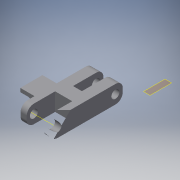
# Autodesk Inventor part: lever2
Saved by Autodesk Inventor 2016 (Build 200138000, 138)
## iProperties
Created: 2015-09-30
Part Number: lever2
Material: Generic
Document SubType Name: Modeling
Designer: Jesse Stevenson
Density: 1 g/cm^3
Appearance: Default
Author: Jesse Stevenson
Autodesk Inventor part; units mm, degrees
ref_plane "YZ Plane" through (0, 0, 0) normal (1, 0, 0) x (0, 1, 0)
ref_plane "XZ Plane" through (0, 0, 0) normal (0, 1, 0) x (-1, 0, 0)
ref_plane "XY Plane" through (0, 0, 0) normal (0, 0, 1) x (1, 0, 0)
ref_plane "Work Plane1" through (8.001, 26.0985, -18.0717) normal (0, 1, 0) x (0, 0, -1)
sketch "Sketch1" plane through (8.001, 26.0985, -18.0717) normal (0, 1, 0) x (0, 0, -1)
  line L0 (-43.7282, -1.4601) -> (-43.7282, -1.8842)
  line L1 (-43.7282, -1.8842) -> (-9.3098, -1.8842)
  line L2 (-9.3098, -1.8842) -> (-9.3098, 2.815)
  line L3 (-43.7282, 11.0271) -> (-43.7282, 11.4512)
  line L4 (-43.7282, 11.4512) -> (-9.3098, 11.4512)
  line L5 (-9.3098, 11.4512) -> (-9.3098, 6.752)
  line L6 (-43.7282, -1.4601) -> (-43.7282, 11.0271)
  line L7 (-9.3098, 2.815) -> (-25.0363, 2.815)
  line L8 (-25.0363, 2.815) -> (-25.0363, 6.752)
  line L9 (-25.0363, 6.752) -> (-9.3098, 6.752)
  line L10 (-18.0537, 2.815) -> (-18.0537, -1.8842) construction
  line L11 (-18.0537, 6.752) -> (-18.0537, 11.4512) construction
  line L12 (-16.6851, 3.45) -> (-16.6851, 6.117) construction
  line L13 (-16.6851, 3.45) -> (-12.9069, 3.45) construction
  line L14 (-12.9069, 3.45) -> (-12.9069, 6.117) construction
  line L15 (-12.9069, 6.117) -> (-16.6851, 6.117) construction
  point P0 (-18.0717, 8.001)
  dimension "d19" = 0.635
  dimension "d20" = 0.635
  constraints: 24 end point, 6 point on line, 4 collinear, 3 parallel, 3 perpendicular, 2 horizontal
  measures "d19" distance between parallel lines of L7 L13
  measures "d20" distance between parallel lines of L9 L15
extrude "Extrusion1" add sketch "Sketch1" along normal blind 7.9375
sketch "Sketch2" plane through (9.8852, 26.0985, 25.6565) normal (1, 0, 0) x (0, 0, -1)
  line L0 (34.4184, 0) -> (0, 0) construction
  line L1 (34.4184, 0) -> (34.4184, 7.9375) construction
  line L2 (0, 7.9375) -> (34.4184, 7.9375) construction
  line L3 (0, 0) -> (0, 7.9375) construction
  line L4 (34.4184, 0) -> (34.4184, 7.9375) construction
  line L5 (34.4184, 3.9687) -> (0, 3.9687) construction
  line L6 (34.4184, 0) -> (0, 0) construction
  line L7 (28.9311, 0) -> (28.9311, 7.9375) construction
  line L8 (34.4184, 7.9375) -> (14.8298, 7.9375) construction
  circle A0 centre (28.9311, 3.9687) radius 1.7859
  point P0 (25.6565, -26.0985)
  dimension "d8" = 3.5719
  constraints: 4 end point, 3 midpoint, 3 point on line, 1 centre point, 1 perpendicular
  measures "d8" diameter of A0
extrude "Extrusion2" cut sketch "Sketch2" against normal through all
fillet "Fillet1" radius 3.175 2 edges at (3.2175, 34.036, 25.6565) (3.2175, 26.0985, 25.6565)
sketch "Sketch3" plane through (9.8852, 26.0985, -8.7619) normal (1, 0, 0) x (0, 0, -1)
  circle A0 centre (-5.4873, 3.9688) radius 1.7859 projected
  line L0 (0, 0) -> (-31.2434, 0) projected
  line L1 (0, 0) -> (0, 7.9375) projected
  line L2 (-31.2434, 7.9375) -> (0, 7.9375) projected
  line L3 (-34.4184, 3.175) -> (-34.4184, 4.7625) projected
  line L4 (-31.2434, 3.175) -> (-31.2434, 4.7625) construction
  circle A1 centre (-31.2434, 3.9687) radius 1.7859
  arc A2 (-34.4184, 3.175) -> (-31.2434, 0) centre (-31.2434, 3.175) ccw projected
  arc A3 (-31.2434, 7.9375) -> (-34.4184, 4.7625) centre (-31.2434, 4.7625) ccw projected
  point P0 (-8.7619, -26.0985)
  dimension "d7" = 3.5719
  constraints: 2 end point, 1 centre point, 1 midpoint, 1 vertical
  measures "d7" diameter of A1
extrude "Extrusion3" cut sketch "Sketch3" against normal through all contours A1
sketch "Sketch5" plane through (9.8852, 26.0985, -8.7619) normal (1, 0, 0) x (0, 0, -1)
  circle A0 centre (-31.2434, 3.9688) radius 1.7859 construction
  circle A1 centre (-5.4873, 3.9688) radius 1.7859 construction
  line L0 (0, 0) -> (-31.2434, 0) construction
  line L1 (0, 0) -> (0, 7.9375) construction
  line L2 (-31.2434, 7.9375) -> (0, 7.9375) construction
  line L3 (-34.4184, 3.175) -> (-34.4184, 4.7625) construction
  line L4 (-15.9544, 0) -> (0, 0) projected
  line L5 (-2.2351, 0) -> (-2.2351, 7.9375)
  line L6 (-15.9544, 7.9375) -> (0, 7.9375) projected
  line L7 (-2.2351, 0) -> (-8.7527, 0)
  line L8 (-34.4184, 7.9375) -> (0, 7.9375) projected
  line L9 (-2.2351, 0) -> (0, 0)
  line L10 (0, 0) -> (0, 7.9375)
  line L11 (0, 7.9375) -> (-2.2351, 7.9375)
  line L12 (-2.2351, 7.9375) -> (-2.2351, 0)
  arc A2 (-34.4184, 3.175) -> (-31.2434, 0) centre (-31.2434, 3.175) ccw projected
  arc A3 (-31.2434, 7.9375) -> (-34.4184, 4.7625) centre (-31.2434, 4.7625) ccw projected
  point P0 (-8.7619, -26.0985)
  constraints: 12 end point, 3 point on line, 2 parallel, 2 perpendicular, 1 horizontal
extrude "Extrusion4" cut sketch "Sketch5" against normal through all
fillet "Fillet2" radius 3.175 4 edges at (7.5356, 34.036, -6.5269) (-1.1006, 34.036, -6.5269) (7.5356, 26.0985, -6.5269) (-1.1006, 26.0985, -6.5269)
sketch "Sketch6" plane through (8.001, 26.0985, -18.0717) normal (0, -1, 0) x (1, 0, 0)
  line L0 (-1.7153, 46.6729) -> (-1.7153, 39.3669) construction
  line L1 (-8.0653, 39.3669) -> (-8.0653, 46.6729) construction
  line L2 (-1.0803, 47.2656) -> (-1.0803, 39.3486) construction
  line L3 (-8.7003, 39.3486) -> (-8.7003, 42.6343) construction
  line L4 (-1.0803, 47.2656) -> (-8.7003, 47.2656)
  line L5 (-8.7003, 47.2656) -> (-8.7003, 31.0791)
  line L6 (-8.7003, 31.0791) -> (-1.0803, 31.0791)
  line L7 (-1.0803, 31.0791) -> (-1.0803, 47.2656)
  point P0 (-8.001, 18.0717)
  dimension "d12" = 0.635
  dimension "d13" = 0.635
  constraints: 16 end point, 4 parallel, 1 horizontal, 1 perpendicular
  measures "d12" distance between parallel lines of L0 L2
  measures "d13" distance between parallel lines of L1 L3
extrude "Extrusion5" cut sketch "Sketch6" against normal through all
sketch "Sketch8" plane through (-3.4502, 29.2735, 25.6565) normal (-1, 0, 0) x (0, 0, 1)
  arc A0 (-32.1833, 0) -> (-29.0083, -3.175) centre (-29.0083, 0) ccw construction
  line L0 (-3.175, -3.175) -> (-29.0083, -3.175) construction
  arc A1 (-3.175, -3.175) -> (0, 0) centre (-3.175, 0) ccw construction
  line L1 (0, 0) -> (0, 1.5875) construction
  arc A2 (0, 1.5875) -> (-3.175, 4.7625) centre (-3.175, 1.5875) ccw construction
  line L2 (-29.0083, 4.7625) -> (-3.175, 4.7625) construction
  arc A3 (-29.0083, 4.7625) -> (-32.1833, 1.5875) centre (-29.0083, 1.5875) ccw construction
  line L3 (-32.1833, 1.5875) -> (-32.1833, 0) construction
  circle A4 centre (-3.175, 0.7938) radius 1.7859 construction
  circle A5 centre (-28.9311, 0.7938) radius 1.7859 construction
  line L4 (-3.175, 4.7625) -> (-29.0083, 4.7625) projected
  line L5 (-6.2153, 4.7625) -> (-16.0917, 4.7625)
  line L6 (-16.0917, 4.7625) -> (-16.0917, 3.1144)
  line L7 (-16.0917, 3.1144) -> (-6.2153, 3.1144)
  line L8 (-6.2153, 3.1144) -> (-6.2153, 4.7625)
  point P0 (-25.6565, -29.2735)
  constraints: 8 end point, 2 parallel, 1 horizontal, 1 perpendicular, 1 point on line
extrude "Extrusion7" add sketch "Sketch8" along normal blind 6.35
fillet "Fillet3" radius 3.175 1 edges at (-3.4502, 32.3879, 14.503)
body "Solid1"
